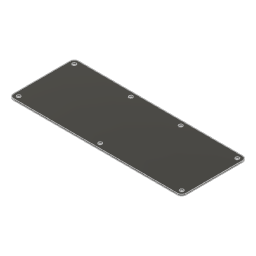
Bottom Panel Full (Autodesk Fusion 360 design; units mm, degrees)
Autodesk Fusion 360 part; units mm, degrees
sketch "Sketch1" plane through (0, 0, 0) normal (0, 0, 1) x (1, 0, 0)
  circle A0 centre (53, 59) radius 3.75
  arc A1 (174, -69) -> (183, -60) centre (174, -60) ccw
  line L0 (183, 60) -> (183, -60)
  arc A2 (183, 60) -> (174, 69) centre (174, 60) ccw
  arc A3 (-183, -60) -> (-174, -69) centre (-174, -60) ccw
  circle A4 centre (173, -59) radius 3.75
  line L1 (-183, -60) -> (-183, 60)
  arc A5 (-174, 69) -> (-183, 60) centre (-174, 60) ccw
  line L2 (174, -69) -> (-174, -69)
  circle A6 centre (0, -59) radius 3.75
  circle A7 centre (-173, 59) radius 3.75
  circle A8 centre (173, 59) radius 3.75
  circle A9 centre (-53, 59) radius 3.75
  circle A10 centre (-173, -59) radius 3.75
  line L3 (-174, 69) -> (174, 69)
  dimension "d1" = 9
  dimension "d25" = 7.5
  dimension "d26" = 7.5
  dimension "d27" = 7.5
  dimension "d28" = 7.5
  dimension "d29" = 7.5
  dimension "d35" = 7.5
  dimension "d9" = 7.5
  constraint horizontal L2
  constraint vertical L0
  constraint vertical L1
  constraint tangent L1 A5
  constraint tangent A3 L1
  constraint tangent A3 L2
  constraint equal A3 A5
  constraint tangent A1 L2
  constraint tangent A1 L0
  constraint equal A1 A5
  constraint tangent L0 A2
  constraint equal A2 A5
  constraint tangent A2 L3
  measures "d1" radius of A5
  measures "d25" diameter of A7
  measures "d26" diameter of A9
  measures "d27" diameter of A0
  measures "d28" diameter of A8
  measures "d29" diameter of A4
  measures "d35" diameter of A10
  measures "d9" diameter of A6
extrude "Extrude1" add sketch "Sketch1" along normal blind 3
